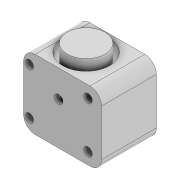
# Autodesk Inventor part: Hinge_p1
Saved by Autodesk Inventor 2022 (Build 260153000, 153)
## iProperties
Created: 2022-07-09
Part Number: Hinge_p1
Material: Generic
Document SubType Name: Modeling
Designer: dell
Density: 1 g/cm^3
Appearance: Default
Author: dell
Autodesk Inventor part; units mm, degrees
ref_plane "YZ Plane" through (0, 0, 0) normal (1, 0, 0) x (0, 1, 0)
ref_plane "XZ Plane" through (0, 0, 0) normal (0, 1, 0) x (-1, 0, 0)
ref_plane "XY Plane" through (0, 0, 0) normal (0, 0, 1) x (1, 0, 0)
sketch "Sketch1" plane through (0, 0, 0) normal (0, 1, 0) x (-1, 0, 0)
  circle A0 centre (0, 0) radius 4.9
  circle A1 centre (0, 0) radius 6.1
  line L0 (-9.1, 7.1) -> (9.1, 7.1)
  line L1 (9.1, 7.1) -> (9.1, -7.1)
  line L2 (9.1, -7.1) -> (-9.1, -7.1)
  line L3 (-9.1, -7.1) -> (-9.1, 7.1)
  dimension "d0" = 9.8
  dimension "d1" = 12.2
  dimension "d36" = 1
  dimension "d37" = 1
  dimension "d38" = 3
  dimension "d39" = 3
  constraints: 8 end point, 2 centre point, 2 coincident, 2 parallel, 1 horizontal, 1 perpendicular
  measures "d0" diameter of A0
  measures "d1" diameter of A1
  measures "d36" distance edge to line of A1 L0
  measures "d37" distance edge to line of A1 L2
  measures "d38" distance edge to line of A1 L1
  measures "d39" distance edge to line of A1 L3
extrude "Extrusion1" add sketch "Sketch1" along normal blind 15
sketch "Sketch2" plane through (0, 15, 0) normal (0, 1, 0) x (1, 0, 0)
  circle A0 centre (0, 0) radius 4.9 projected
extrude "Extrusion2" add sketch "Sketch2" along normal blind 2
sketch "Sketch3" plane through (0, 0, 0) normal (0, -1, 0) x (1, 0, 0)
  circle A0 centre (0, 0) radius 6.1 projected
  line L0 (9.1, -7.1) -> (-9.1, -7.1) projected
  line L1 (-9.1, -7.1) -> (-9.1, 7.1) projected
  line L2 (-9.1, 7.1) -> (9.1, 7.1) projected
  line L3 (9.1, 7.1) -> (9.1, -7.1) projected
  circle A1 centre (0, 0) radius 6.1 projected
extrude "Extrusion3" add sketch "Sketch3" along normal blind 3 contours A0 | L0 L1 L2 L3
sketch "Sketch8" plane through (-9.1, 0, 7.1) normal (0, 0, 1) x (1, 0, 0)
  circle A0 centre (16.7, 0) radius 1.1
  circle A1 centre (16.7, 12) radius 1.1
  circle A2 centre (1.5, 0) radius 1.1
  circle A3 centre (1.5, 12) radius 1.1
  line L0 (3, 15) -> (15.2, 15) projected
  line L1 (3, 0) -> (15.2, 0) projected
  line L2 (3, 15) -> (3, 0) projected
  line L3 (15.2, 15) -> (15.2, 0) projected
  line L4 (18.2, 0) -> (18.2, 15) projected
  line L5 (0, 0) -> (0, 15) projected
  line L6 (0, 15) -> (18.2, 15) projected
  line L7 (0, 0) -> (18.2, 0) projected
  point P0 (9.1, 0)
  dimension "d40" = 2.2
  dimension "d41" = 2.2
  dimension "d42" = 2.2
  dimension "d43" = 2.2
  dimension "d44" = 3
  dimension "d45" = 3
  dimension "d46" = 1.5
  dimension "d47" = 1.5
  dimension "d48" = 1.5
  dimension "d49" = 1.5
  dimension "d50" = 3
  dimension "d51" = 0
  dimension "d52" = 0
  dimension "d53" = 3
  constraints: 4 centre point
  measures "d40" diameter of A0
  measures "d41" diameter of A1
  measures "d42" diameter of A2
  measures "d43" diameter of A3
  measures "d44" distance between parallel lines of L3 L4
  measures "d45" distance between parallel lines of L5 L2
  measures "d46" distance from line of L3 A1.centre
  measures "d47" distance from line of L3 A0.centre
  measures "d48" distance from line of L2 A2.centre
  measures "d49" distance from line of L2 A3.centre
  measures "d50" distance from line of L6 A1.centre
  measures "d51" distance from line of L7 A0.centre
  measures "d52" distance from line of L7 A2.centre
  measures "d53" distance from line of L6 A3.centre
extrude "Extrusion8" cut sketch "Sketch8" against normal blind 100 contours L7 A0 | A0 L7 | L7 A2 | A2 L7 | A1 | A3
sketch "Sketch9" plane through (9.1, 15, 7.1) normal (1, 0, 0) x (0, 0, -1)
  line L0 (14.2, 0) -> (14.2, -18) projected
  line L1 (0, 0) -> (14.2, 0) projected
  line L2 (0, -18) -> (0, 0) projected
  line L3 (14.2, -18) -> (0, -18) projected
  point P0 (7.1, -15)
extrude "Extrusion9" add sketch "Sketch9" along normal blind 2
fillet "Fillet8" radius 3 4 edges at (-9.1, -3, 0) (11.1, -3, 0) (11.1, 15, 0) (-9.1, 15, 0)
sketch "Sketch10" plane through (-6.1, -3, 7.1) normal (0, 0, 1) x (1, 0, 0)
  line L0 (0, 3) -> (12.2, 3) projected
  line L1 (0, 18) -> (0, 3) projected
  line L2 (12.2, 18) -> (12.2, 3) projected
  line L3 (0, 18) -> (12.2, 18) projected
  circle A0 centre (6.1, 11) radius 1.1
  point P0 (6.1, 3)
  point P1 (6.1, 3)
  dimension "d59" = 2.2
  dimension "d60" = 8
  constraints: 1 centre point, 1 midpoint, 1 vertical alignment
  measures "d59" diameter of A0
  measures "d60" distance from line of L0 A0.centre
extrude "Extrusion10" cut sketch "Sketch10" against normal blind 100 contours A0
equation "\"d46\" = 0.5 * d44"
equation "\"d47\" = 0.5 * d44"
equation "\"d48\" = 0.5 * d45"
equation "\"d49\" = 0.5 * d45"
body "Solid1"
